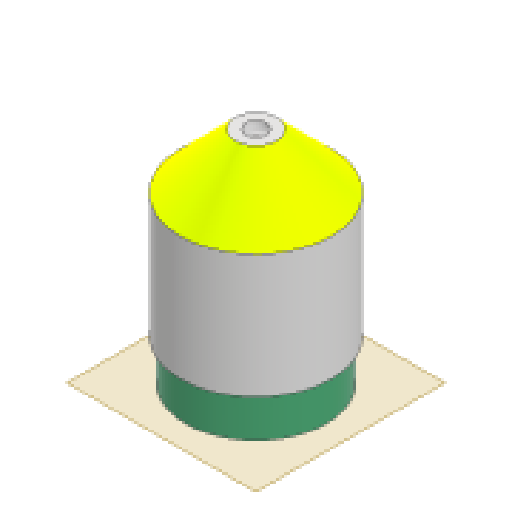
# Autodesk Inventor part: Objective_placeholder_V2
Saved by Autodesk Inventor 2023 (Build 270158000, 158)
## iProperties
Created: 2021-07-06
Part Number: Objective_placeholder_V2
Material: Generic
Document SubType Name: Modeling
Designer: CDT
Density: 1 g/cm^3
Appearance: Default
Author: CDT
Autodesk Inventor part; units mm, degrees
ref_plane "YZ Plane" through (0, 0, 0) normal (1, 0, 0) x (0, 1, 0)
ref_plane "XZ Plane" through (0, 0, 0) normal (0, 1, 0) x (-1, 0, 0)
ref_plane "XY Plane" through (0, 0, 0) normal (0, 0, 1) x (1, 0, 0)
ref_plane "Work Plane1" through (-149.1228, -3.9521, -261.8445) normal (0, 1, 0) x (1, 0, 0)
sketch "Sketch1" plane through (-149.1228, -3.9521, -261.8445) normal (0, 1, 0) x (1, 0, 0)
  circle A0 centre (0, 0) radius 11
  point P0 (149.1228, -261.8445)
  dimension "d0" = 22
  constraints: 1 centre point
  measures "d0" diameter of A0
extrude "Extrusion1" add sketch "Sketch1" along normal blind 32
sketch "Sketch2" plane through (-149.1228, 28.0479, -261.8445) normal (0, 1, 0) x (1, 0, 0)
  circle A0 centre (0, 0) radius 1
  point P0 (149.1228, -261.8445)
  dimension "d3" = 2
  constraints: 1 centre point
  measures "d3" diameter of A0
extrude "Extrusion2" [suppressed]
sketch "Sketch3" plane through (-149.1228, -3.9521, -261.8445) normal (0, -1, 0) x (1, 0, 0)
  circle A0 centre (0, 0) radius 11
  circle A1 centre (0, 0) radius 10.25
  point P0 (149.1228, 261.8445)
  dimension "d6" = 22
  dimension "d7" = 20.5
  constraints: 2 centre point, 1 coincident
  measures "d6" diameter of A0
  measures "d7" diameter of A1
extrude "Extrusion3" cut sketch "Sketch3" against normal blind 6
chamfer "Chamfer1" distance 8 angle 45 1 edges at (-160.1228, 28.0479, -261.8445)
sketch "Sketch4" plane through (-149.1228, 28.0479, -261.8445) normal (0, 1, 0) x (1, 0, 0)
  circle A0 centre (0, 0) radius 11 projected
  circle A1 centre (0, 0) radius 1.5
  point P0 (149.1228, -261.8445)
  dimension "d13" = 3
  constraints: 1 centre point, 1 coincident
  measures "d13" diameter of A1
extrude "Extrusion4" cut sketch "Sketch4" against normal blind 1 contours A1
fillet "Fillet1" radius 1 1 edges at (-150.6228, 27.0479, -261.8445)
body "Solid1"
